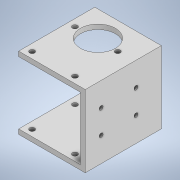
# Autodesk Inventor part: サーボモータ固定２軸
Saved by Autodesk Inventor 2022 (Build 260153000, 153)
## iProperties
Created: 2022-11-23
Part Number: サーボモータ固定２軸
Material: 一般
Document SubType Name: Modeling
Designer: tdn82
Density: 1 g/cm^3
Appearance: 既定
Author: tdn82
Autodesk Inventor part; units mm, degrees
ref_plane "YZ Plane" through (0, 0, 0) normal (1, 0, 0) x (0, 1, 0)
ref_plane "XZ Plane" through (0, 0, 0) normal (0, 1, 0) x (-1, 0, 0)
ref_plane "XY Plane" through (0, 0, 0) normal (0, 0, 1) x (1, 0, 0)
sketch "スケッチ1" plane through (0, 0, 0) normal (0, 1, 0) x (-1, 0, 0)
  line L0 (0, 0) -> (-42, 0)
  line L1 (-42, 0) -> (-42, -48)
  line L2 (-42, -48) -> (0, -48)
  line L3 (0, -48) -> (0, 0)
  dimension "d0" = 48
  dimension "d1" = 42
  constraints: 8 end point, 2 parallel, 1 horizontal, 1 perpendicular
  measures "d0" distance of L0.end L1.end
  measures "d1" distance of L1.end L2.end
extrude "押し出し1" add sketch "スケッチ1" along normal blind 45.5
sketch "スケッチ2" plane through (42, 0, -48) normal (0, 0, -1) x (-1, 0, 0)
  line L0 (3, 42.5) -> (59.072, 42.5)
  line L1 (59.072, 42.5) -> (59.072, 3)
  line L2 (59.072, 3) -> (3, 3)
  line L3 (3, 3) -> (3, 42.5)
  line L4 (0, 45.5) -> (42, 45.5) projected
  line L5 (0, 0) -> (42, 0) projected
  line L6 (0, 0) -> (0, 45.5) projected
  dimension "d4" = 39.5
  dimension "d6" = 3
  dimension "d7" = 3
  constraints: 8 end point, 2 parallel, 1 horizontal, 1 perpendicular
  measures "d4" distance of L2.end L0.start
  measures "d6" distance between parallel lines of L2 L5
  measures "d7" distance between parallel lines of L6 L3
extrude "押し出し2" cut sketch "スケッチ2" against normal blind 100
sketch "スケッチ3" plane through (0, 45.5, 0) normal (0, 1, 0) x (1, 0, 0)
  line L0 (42, 48) -> (0, 48) projected
  line L1 (42, 0) -> (42, 48) projected
  point P0 (0, 0)
  point P1 (18, 32)
  dimension "d10" = 16
  dimension "d11" = 24
  measures "d10" distance from line of L0 point (18, 32)
  measures "d11" distance from line of L1 point (18, 32)
hole "穴1" at (18, 45.5, -32) direction (0, -1, 0) diameter 22 depth 3 tip angle 118
sketch "スケッチ4" plane through (0, 45.5, 0) normal (0, 1, 0) x (1, 0, 0)
  line L0 (0, 0) -> (42, 0) projected
  line L1 (42, 0) -> (42, 48) projected
  point P0 (31.5, 4)
  point P1 (31.5, 31)
  point P2 (4.5, 4)
  point P3 (4.5, 31)
  point P4 (4.5, 4)
  dimension "d19" = 4
  dimension "d20" = 10.5
  dimension "d23" = 27
  dimension "d26" = 27
  constraints: 1 coincident, 1 horizontal, 1 vertical, 3 other
  measures "d19" distance from line of L0 point (31.5, 4)
  measures "d20" distance from line of L1 point (31.5, 4)
  measures "d23" distance of point (31.5, 4) point (31.5, 31)
  measures "d26" distance of point (31.5, 4) point (4.5, 4)
hole "穴2" at (31.5, 45.5, -4) at (31.5, 45.5, -31) at (4.5, 45.5, -31) at (4.5, 45.5, -4) direction (0, -1, 0) diameter 3.2 end through all
sketch "スケッチ5" plane through (0, 0, 0) normal (0, -1, 0) x (1, 0, 0)
  line L0 (0, -48) -> (0, 0) projected
  line L1 (42, -48) -> (0, -48) projected
  point P0 (18, -32)
  dimension "d36" = 18
  dimension "d37" = 16
  measures "d36" distance from line of L0 point (18, -32)
  measures "d37" distance from line of L1 point (18, -32)
hole "穴3" at (18, 0, -32) direction (0, 1, 0) diameter 13 end through all
sketch "スケッチ6" plane through (42, 0, 0) normal (1, 0, 0) x (0, 0, -1)
  line L0 (0, 45.5) -> (48, 45.5) projected
  line L1 (0, 0) -> (0, 45.5) projected
  point P0 (10, 30.5)
  point P1 (32, 30.5)
  point P2 (10, 15.5)
  point P3 (32, 15.5)
  dimension "d45" = 15
  dimension "d46" = 10
  dimension "d49" = 22
  dimension "d52" = 15
  constraints: 1 horizontal, 1 vertical, 3 other
  measures "d45" distance from line of point (10, 30.5) L0
  measures "d46" distance from line of L1 point (10, 30.5)
  measures "d49" distance of point (10, 30.5) point (32, 30.5)
  measures "d52" distance of point (10, 30.5) point (10, 15.5)
hole "穴4" at (42, 30.5, -10) at (42, 30.5, -32) at (42, 15.5, -10) at (42, 15.5, -32) direction (-1, 0, 0) diameter 2.5 end through all
